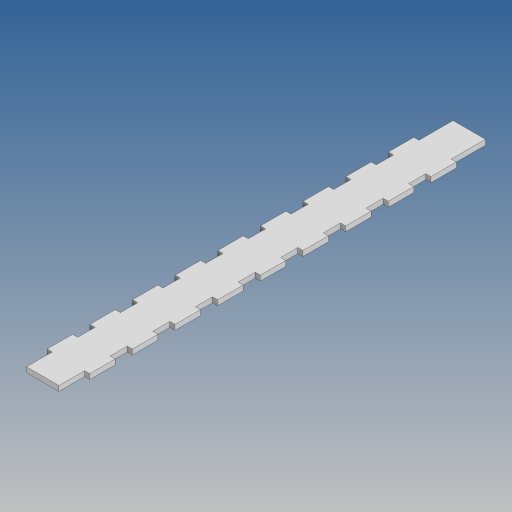
# Autodesk Inventor part: Pieza5
Saved by Autodesk Inventor 2024 (Build 280153000, 153)
## iProperties
Created: 2024-05-31
Part Number: Pieza5
Material: Genérico
Document SubType Name: Modeling
Designer: Pablo
Density: 1 g/cm^3
Appearance: Valor por defecto
Author: Pablo
Autodesk Inventor part; units mm, degrees
ref_plane "YZ Plane" through (0, 0, 0) normal (1, 0, 0) x (0, 1, 0)
ref_plane "XZ Plane" through (0, 0, 0) normal (0, 1, 0) x (-1, 0, 0)
ref_plane "XY Plane" through (0, 0, 0) normal (0, 0, 1) x (1, 0, 0)
sketch "Boceto1" plane through (0, 0, 0) normal (0, 1, 0) x (-1, 0, 0)
  line L0 (0, 0) -> (19, 0)
  line L1 (19, 0) -> (19, -250)
  line L2 (19, -250) -> (0, -250)
  line L3 (0, -250) -> (0, 0)
  line L4 (9.5, 0) -> (9.5, -250) construction
  line L5 (19, -125) -> (0, -125) construction
  line L6 (19, -15) -> (22, -15)
  line L7 (22, -15) -> (22, -30)
  line L8 (22, -30) -> (19, -30)
  line L9 (19, -30) -> (19, -15)
  line L10 (19, -40) -> (22, -40)
  line L11 (22, -40) -> (22, -55)
  line L12 (22, -55) -> (19, -55)
  line L13 (19, -55) -> (19, -40)
  line L14 (19, -65) -> (22, -65)
  line L15 (22, -65) -> (22, -80)
  line L16 (22, -80) -> (19, -80)
  line L17 (19, -80) -> (19, -65)
  line L18 (19, -90) -> (22, -90)
  line L19 (22, -90) -> (22, -105)
  line L20 (22, -105) -> (19, -105)
  line L21 (19, -105) -> (19, -90)
  line L22 (19, -115) -> (22, -115)
  line L23 (22, -115) -> (22, -130)
  line L24 (22, -130) -> (19, -130)
  line L25 (19, -130) -> (19, -115)
  line L26 (19, -140) -> (22, -140)
  line L27 (22, -140) -> (22, -155)
  line L28 (22, -155) -> (19, -155)
  line L29 (19, -155) -> (19, -140)
  line L30 (19, -165) -> (22, -165)
  line L31 (22, -165) -> (22, -180)
  line L32 (22, -180) -> (19, -180)
  line L33 (19, -180) -> (19, -165)
  line L34 (19, -190) -> (22, -190)
  line L35 (22, -190) -> (22, -205)
  line L36 (22, -205) -> (19, -205)
  line L37 (19, -205) -> (19, -190)
  line L38 (19, -215) -> (22, -215)
  line L39 (22, -215) -> (22, -230)
  line L40 (22, -230) -> (19, -230)
  line L41 (19, -230) -> (19, -215)
  line L42 (0, -15) -> (-3, -15)
  line L43 (-3, -15) -> (-3, -30)
  line L44 (-3, -30) -> (0, -30)
  line L45 (0, -30) -> (0, -15)
  line L46 (0, -40) -> (-3, -40)
  line L47 (-3, -40) -> (-3, -55)
  line L48 (-3, -55) -> (0, -55)
  line L49 (0, -55) -> (0, -40)
  line L50 (0, -65) -> (-3, -65)
  line L51 (-3, -65) -> (-3, -80)
  line L52 (-3, -80) -> (0, -80)
  line L53 (0, -80) -> (0, -65)
  line L54 (0, -90) -> (-3, -90)
  line L55 (-3, -90) -> (-3, -105)
  line L56 (-3, -105) -> (0, -105)
  line L57 (0, -105) -> (0, -90)
  line L58 (0, -115) -> (-3, -115)
  line L59 (-3, -115) -> (-3, -130)
  line L60 (-3, -130) -> (0, -130)
  line L61 (0, -130) -> (0, -115)
  line L62 (0, -140) -> (-3, -140)
  line L63 (-3, -140) -> (-3, -155)
  line L64 (-3, -155) -> (0, -155)
  line L65 (0, -155) -> (0, -140)
  line L66 (0, -165) -> (-3, -165)
  line L67 (-3, -165) -> (-3, -180)
  line L68 (-3, -180) -> (0, -180)
  line L69 (0, -180) -> (0, -165)
  line L70 (0, -190) -> (-3, -190)
  line L71 (-3, -190) -> (-3, -205)
  line L72 (-3, -205) -> (0, -205)
  line L73 (0, -205) -> (0, -190)
  line L74 (0, -215) -> (-3, -215)
  line L75 (-3, -215) -> (-3, -230)
  line L76 (-3, -230) -> (0, -230)
  line L77 (0, -230) -> (0, -215)
  point P0 (20.5, -15)
  point P1 (20.5, -40)
  point P2 (20.5, -65)
  point P3 (20.5, -90)
  point P4 (20.5, -115)
  point P5 (20.5, -140)
  point P6 (20.5, -165)
  point P7 (20.5, -190)
  point P8 (20.5, -215)
  point P9 (44, 0)
  point P10 (-1.5, -15)
  point P11 (-1.5, -40)
  point P12 (-1.5, -65)
  point P13 (-1.5, -90)
  point P14 (-1.5, -115)
  point P15 (-1.5, -140)
  point P16 (-1.5, -165)
  point P17 (-1.5, -190)
  point P18 (-1.5, -215)
  point P19 (19, -230)
  point P20 (19, -215)
  point P21 (19, -205)
  point P22 (19, -190)
  point P23 (19, -180)
  point P24 (19, -165)
  point P25 (19, -155)
  point P26 (19, -140)
  point P27 (19, -130)
  point P28 (19, -115)
  point P29 (19, -105)
  point P30 (19, -90)
  point P31 (19, -80)
  point P32 (19, -65)
  point P33 (19, -55)
  point P34 (19, -40)
  point P35 (19, -30)
  dimension "d0" = 19
  dimension "d1" = 250
  dimension "d5" = 3
  dimension "d6" = 15
  dimension "d7" = 15
  dimension "d10" = 25
  constraints: 152 end point, 45 symmetric about line, 40 vertical alignment, 19 parallel, 16 collinear, 3 horizontal, 3 midpoint, 1 perpendicular, 1 point on line, 9 other
  measures "d0" distance of L2.start L2.end
  measures "d1" distance of L0.end L2.start
  measures "d5" distance of L7.end L8.end
  measures "d6" distance of L6.end L7.end
  measures "d7" distance from line of point (20.5, -15) L0
  measures "d10" distance of L6.start L10.start
extrude "Extrusión1" add sketch "Boceto1" along normal blind 3
